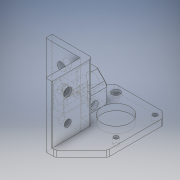
# Autodesk Inventor part: XY Stepper Mount 1.0
Saved by Autodesk Inventor 2016 (Build 200138000, 138)
## iProperties
Created: 2016-12-30
Part Number: XY Stepper Mount 1.0
Material: PET Plastic
Document SubType Name: Modeling
Designer: Scott
Density: 1.541 g/cm^3
Appearance: Gunmetal
Author: Scott
Autodesk Inventor part; units mm, degrees
ref_plane "YZ Plane" through (0, 0, 0) normal (1, 0, 0) x (0, 1, 0)
ref_plane "XZ Plane" through (0, 0, 0) normal (0, 1, 0) x (-1, 0, 0)
ref_plane "XY Plane" through (0, 0, 0) normal (0, 0, 1) x (1, 0, 0)
sketch "Sketch1" plane through (0, 0, 0) normal (0, 0, 1) x (1, 0, 0)
  line L0 (-20.5, 21) -> (21, 21)
  line L1 (21, 21) -> (21, -27.5)
  circle A0 centre (0, 0) radius 11.2
  line L2 (-35, -21) -> (-7.5, -21)
  line L3 (-7.5, -21) -> (-7.5, -48.5)
  line L4 (-7.5, -48.5) -> (0, -48.5)
  line L5 (0, -48.5) -> (21, -27.5)
  line L6 (-35, -21) -> (-35, 6.5)
  line L7 (-35, 6.5) -> (-20.5, 21)
  dimension "d0" = 21
  dimension "d1" = 21
  dimension "d3" = 22.4
  dimension "d4" = 21
  dimension "d5" = 7.5
  dimension "d6" = 27.5
  dimension "d7" = 27.5
  dimension "d8" = 135
  dimension "d9" = 135
  dimension "d10" = 7.5
  dimension "d11" = 27.5
  constraints: 16 end point, 3 horizontal, 2 perpendicular, 1 centre point, 1 coincident, 1 vertical
  measures "d0" distance from line of point (0, 0) L0
  measures "d1" distance from line of point (0, 0) L1
  measures "d3" diameter of A0
  measures "d4" distance from line of A0.centre L2
  measures "d5" distance from line of point (0, 0) L3
  measures "d6" distance of L2.end L3.end
  measures "d7" distance of L2.start L2.end
  measures "d8" angle of L7 L0
  measures "d9" angle of L5 L1
  measures "d10" distance of L3.end L4.end
  measures "d11" distance from line of L2 L6.end
extrude "Extrusion1" add sketch "Sketch1" along normal blind 5
chamfer "Chamfer1" distance 5 angle 45 1 edges at (21, 21, 2.5)
sketch "Sketch2" plane through (0, 0, 5) normal (0, 0, 1) x (1, 0, 0)
  line L0 (-35, -21) -> (-7.5, -21) projected
  line L1 (-7.5, -21) -> (-7.5, -48.5) projected
  line L2 (-7.5, -21) -> (-35, -21) projected
  line L3 (-35, -21) -> (-35, -16)
  line L4 (-35, -21) -> (-35, 6.5) projected
  line L5 (-35, -16) -> (-2.5, -16)
  line L6 (-2.5, -16) -> (-2.5, -48.5)
  line L7 (0, -48.5) -> (-7.5, -48.5) projected
  line L8 (-2.5, -48.5) -> (-7.5, -48.5)
  point P0 (0, 0)
  dimension "d17" = 5
  dimension "d18" = 5
  constraints: 8 end point, 2 point on line, 1 collinear, 1 horizontal, 1 perpendicular
  measures "d17" distance of L0.start L3.end
  measures "d18" distance between parallel lines of L1 L6
extrude "Extrusion2" add sketch "Sketch2" along normal blind 46
sketch "Sketch3" plane through (-35, -16, 5) normal (0, 1, 0) x (1, 0, 0)
  line L0 (27.5, 5) -> (27.5, -46)
  line L1 (12.5, -52.473005) -> (12.5, 15.699235) construction
  circle A0 centre (12.5, -32.5) radius 3.2
  circle A1 centre (12.5, -11) radius 5.2
  point P0 (35, 5)
  dimension "d21" = 15
  dimension "d22" = 6.4
  dimension "d23" = 13.5
  dimension "d24" = 10.4
  dimension "d25" = 35
  constraints: 2 centre point, 2 end point, 2 point on line, 1 vertical
  measures "d21" distance between parallel lines of L0 L1
  measures "d22" diameter of A0
  measures "d23" vertical distance of L0.end A0.centre
  measures "d24" diameter of A1
  measures "d25" vertical distance of A1.centre L0.end
extrude "Extrusion3" cut sketch "Sketch3" against normal through all
sketch "Sketch4" plane through (-35, -16, 5) normal (0, 1, 0) x (1, 0, 0)
  circle A0 centre (12.5, -11) radius 5.2
  line L0 (14.5, 0) -> (0, 0)
  circle A1 centre (12.5, -11) radius 5.2
  line L1 (16.642136, -21) -> (8.357864, -21)
  line L2 (0, 0) -> (32.5, 0)
  line L3 (23.8, 0) -> (23.8, -13.842136)
  line L4 (23.8, -13.842136) -> (16.642136, -21)
  line L5 (8.357864, -21) -> (0, -12.642136)
  line L6 (0, 5) -> (0, -46)
  line L7 (0, 0) -> (0, -12.642136)
  line L8 (12.5, -11) -> (12.5, -26.911097) construction
  point P0 (35, 5)
  point P1 (12.5, -21)
  dimension "d28" = 10.4
  dimension "d29" = 10
  dimension "d30" = 135
  dimension "d31" = 135
  dimension "d32" = 10
  dimension "d34" = 11.3
  constraints: 12 end point, 3 point on line, 2 vertical, 1 centre point, 1 coincident, 1 collinear, 1 horizontal, 1 midpoint
  measures "d28" diameter of A1
  measures "d29" distance from line of L1 A0.centre
  measures "d30" angle of L1 L4
  measures "d31" angle of L5 L1
  measures "d32" distance from line of A0.centre L4
  measures "d34" distance from line of L3 A0.centre
extrude "Extrusion4" add sketch "Sketch4" along normal blind 20
sketch "Sketch5" plane through (-2.5, -48.5, 5) normal (1, 0, 0) x (0, 0, -1)
  line L0 (5, 27.5) -> (-46, 27.5) projected
  circle A0 centre (-32.5, 12.5) radius 3.2
  line L1 (-28.5, 27.5) -> (-34.5, 27.5) projected
  circle A1 centre (-11, 12.5) radius 2.7
  line L2 (-46, 0) -> (-46, 32.5) projected
  point P0 (5, 48.5)
  dimension "d46" = 15
  dimension "d48" = 6.4
  dimension "d49" = 13.5
  dimension "d69" = 35
  dimension "d70" = 15
  dimension "d71" = 5.4
  constraints: 2 centre point
  measures "d46" distance from line of L0 A0.centre
  measures "d48" diameter of A0
  measures "d49" horizontal distance of L0.end A0.centre
  measures "d69" distance from line of A1.centre L2
  measures "d70" distance from line of L0 A1.centre
  measures "d71" diameter of A1
extrude "Extrusion5" cut sketch "Sketch5" against normal through all
fillet "Fillet1" radius 2.5 1 edges at (-2.5, -16, 28)
fillet "Fillet2" radius 5 2 edges at (-11.2, -6, 18.8421) (-35, -6, 17.6421)
fillet "Fillet3" radius 2.5 6 edges at (0, -48.5, 2.5) (21, -27.5, 2.5) (21, 16, 2.5) (16, 21, 2.5) (-20.5, 21, 2.5) (-35, 6.5, 2.5)
sketch "Sketch7" plane through (0, 0, 5) normal (0, 0, 1) x (1, 0, 0)
  circle A0 centre (15.5, -15.5) radius 1.75
  circle A1 centre (15.5, 15.5) radius 1.75
  circle A2 centre (-15.5, 15.5) radius 1.75
  circle A3 centre (-3.5, 15.5) radius 1.25
  point P0 (0, 0)
  dimension "d57" = 15.5
  dimension "d58" = 15.5
  dimension "d59" = 15.5
  dimension "d60" = 15.5
  dimension "d61" = 15.5
  dimension "d62" = 15.5
  dimension "d63" = 3.5
  dimension "d66" = 19
  dimension "d67" = 15.5
  dimension "d68" = 2.5
  constraints: 4 centre point, 2 equal radius
  measures "d57" horizontal distance of point (0, 0) A0.centre
  measures "d58" horizontal distance of point (0, 0) A0.centre
  measures "d59" horizontal distance of A1.centre point (0, 0)
  measures "d60" horizontal distance of A1.centre point (0, 0)
  measures "d61" horizontal distance of point (0, 0) A2.centre
  measures "d62" horizontal distance of point (0, 0) A2.centre
  measures "d63" diameter of A2
  measures "d66" distance of A3.centre A1.centre
  measures "d67" vertical distance of point (0, 0) A3.centre
  measures "d68" diameter of A3
extrude "Extrusion7" cut sketch "Sketch7" against normal through all contours A0 | A1 | A2
sketch "Sketch8" plane through (0, 0, 5) normal (0, 0, 1) x (1, 0, 0)
  circle A0 centre (15.5, -15.5) radius 1.75 projected
  circle A1 centre (15.5, 15.5) radius 1.75 projected
  circle A2 centre (-15.5, 15.5) radius 1.75 projected
  circle A3 centre (15.5, -15.5) radius 1.75 projected
  circle A4 centre (15.5, -15.5) radius 3.05
  circle A5 centre (15.5, 15.5) radius 3.05
  circle A6 centre (-15.5, 15.5) radius 1.75 projected
  circle A7 centre (-15.5, 15.5) radius 3.05
  point P0 (0, 0)
  dimension "d72" = 6.1
  dimension "d73" = 6.1
  dimension "d74" = 6.1
  constraints: 3 centre point, 3 coincident
  measures "d72" diameter of A4
  measures "d73" diameter of A5
  measures "d74" diameter of A7
extrude "Extrusion8" cut sketch "Sketch8" against normal blind 2 contours A1 | A7
sketch "Sketch11" plane through (0, 0, 5) normal (0, 0, 1) x (1, 0, 0)
  circle A0 centre (0, 0) radius 11.2 projected
  circle A1 centre (0, 0) radius 11.2
  point P0 (-10.753147, 2.753147)
  point P1 (-11, -2.107131)
  point P2 (-10.354226, 4)
  point P3 (-11, 2.107131)
  constraints: 1 centre point, 1 coincident, 2 other
extrude "Extrusion10" cut sketch "Sketch11" along normal blind 20 draft -15
sketch "Sketch15" plane through (0, 0, 0) normal (0, 0, -1) x (-1, 0, 0)
  line L0 (22.5, 34.9) -> (22.5, -62.4)
  line L1 (35, 4) -> (11.2, 4)
  line L2 (11.2, -16) -> (5, -16)
  line L3 (35, 4) -> (26.5, 4)
  line L4 (25.5, 5) -> (25.5, -16)
  line L5 (25.5, -16) -> (26.5, -16)
  line L6 (18.357864, -16) -> (26.642136, -16)
  line L7 (26.5, -16) -> (26.5, 4)
  line L8 (25.5, 5) -> (35, 5)
  line L9 (35, -21) -> (35, 5.464466)
  line L10 (35, 4) -> (35, 5)
  point P0 (0, 0)
  dimension "d110" = 3
  dimension "d111" = 1
  dimension "d113" = 1
  constraints: 12 end point, 2 perpendicular, 2 point on line, 1 collinear, 1 horizontal, 1 vertical
  measures "d110" distance between parallel lines of L0 L4
  measures "d111" distance between parallel lines of L4 L7
  measures "d113" distance between parallel lines of L8 L1
extrude "Extrusion14" cut sketch "Sketch15" against normal blind 15 contours L4 L8 L9 L1 | L1 L7 L5 L4
sketch "Sketch17" plane through (-26.642136, -16, 26) normal (0, 1, 0) x (1, 0, 0)
  arc A0 (0.142136, 13.32265) -> (1.142136, 14.247352) centre (4.142136, 10) ccw
  line L0 (-6.893398, 6.893398) -> (0, 0)
  arc A1 (-8.357864, 10.428932) -> (-6.893398, 6.893398) centre (-3.357864, 10.428932) ccw
  line L1 (-8.357864, 26) -> (-8.357864, 10.428932)
  line L2 (0.142136, 13.32265) -> (0.142136, 26)
  line L3 (1.142136, 21) -> (1.142136, 14.247352)
  arc A2 (0.142136, 13.32265) -> (1.142136, 14.247352) centre (4.142136, 10) ccw
  line L4 (0.142136, 13.32265) -> (0.142136, 26)
  line L5 (-8.357864, 26) -> (0.142136, 26)
  line L6 (-8.357864, 26) -> (-8.357864, 10.428932)
  arc A3 (-8.357864, 10.428932) -> (-6.893398, 6.893398) centre (-3.357864, 10.428932) ccw
  line L7 (-6.893398, 6.893398) -> (0, 0)
  line L8 (0, 0) -> (8.284271, 0)
  line L9 (8.284271, 0) -> (13.97767, 5.693398)
  arc A4 (13.97767, 5.693398) -> (15.442136, 9.228932) centre (10.442136, 9.228932) ccw
  line L10 (15.442136, 9.228932) -> (15.442136, 21)
  line L11 (1.142136, 21) -> (15.442136, 21)
  line L12 (4.142136, 10) -> (-11.850384, -5.99252) construction
  line L13 (0.46518, 6.323045) -> (-2.928932, 2.928932)
  point P0 (26.642136, 26)
  dimension "d119" = 90
  constraints: 4 end point, 3 point on line, 1 point on circle
  measures "d119" angle of L0 L12
extrude "Extrusion16" cut sketch "Sketch17" along normal blind 1 contours A0 L13 L0 A1 L1 L5 L2
sketch "Sketch18" plane through (-11.2, -16, 5) normal (1, 0, 0) x (0, 0, -1)
  line L0 (-11.771068, 0) -> (-11.771068, 20)
  line L1 (0, 0) -> (-11.771068, 0)
  line L2 (0, 16) -> (0, 0)
  line L3 (0, 20) -> (0, 16)
  line L4 (-11.771068, 20) -> (0, 20)
  line L5 (-11.771068, 0) -> (-11.771068, 20) construction
  line L6 (-11.771068, 10) -> (8.38591, 10) construction
  point P0 (5, 16)
  point P1 (-4, 10)
  dimension "d122" = 4
  constraints: 2 end point, 1 horizontal, 1 midpoint, 1 point on line
  measures "d122" distance from line of L2 point (-4, 10)
hole "Hole3" at (-11.2, -6, 9) direction (-1, 0, 0) diameter 3.5 end through all counterbore diameter 6 counterbore depth 3
hole "Hole4" at (-35, -6, 9) direction (1, 0, 0) diameter 4.7 depth 5 counterbore diameter 5 counterbore depth 1
fillet "Fillet7" radius 0.5 15 edges at (-26.5, 4, 6.3387) (-25.5, 4, 8.3763) (-26.5, -15, 6.3387) (-25.5, -6, 11.7526) (-26.5, -5.5, 12.6774) (-35, 5, 2.5) (-34.6194, -15, 17.4845) (-31.5533, -15, 21.0888) (-35, -15, 7.7855) (-35, 4, 7.7855) (-30.0888, 4, 22.5533) (-34.6194, 4, 17.4845) (-15.5112, 4, 23.1533) (-11.2, 4, 10.8855) (-11.5806, 4, 18.6845)
fillet "Fillet8" radius 0.5 4 edges at (-7.5, -48.5, 25.5) (-2.5, -48.5, 28) (-35, -21, 25.5) (-35, -16, 25.5)
equation "\"d73\" = d72"
equation "\"d74\" = d72"
body "Solid1"
